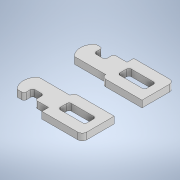
# Autodesk Inventor part: Base_modded
Saved by Autodesk Inventor 2022 (Build 260153000, 153)
## iProperties
Created: 2023-01-30
Part Number: Base_modded
Material: Generic
Document SubType Name: Modeling
Designer: scott
Density: 1 g/cm^3
Appearance: Default
Author: scott
Autodesk Inventor part; units mm, degrees
ref_plane "YZ Plane" through (0, 0, 0) normal (1, 0, 0) x (0, 1, 0)
ref_plane "XZ Plane" through (0, 0, 0) normal (0, 1, 0) x (-1, 0, 0)
ref_plane "XY Plane" through (0, 0, 0) normal (0, 0, 1) x (1, 0, 0)
sketch "Sketch1" plane through (0, 0, 0) normal (0, 1, 0) x (-1, 0, 0)
  line L0 (17.0278, 0) -> (-10.5342, 0)
  line L1 (-10.5342, 0) -> (-10.5342, -20.5)
  line L2 (-10.5342, -20.5) -> (17.0278, -20.5)
  line L3 (17.0278, -20.5) -> (17.0278, 0)
  line L4 (4.9658, -15.846) -> (-7.0342, -15.846)
  line L5 (-7.0342, -15.846) -> (-7.0342, -10.846)
  line L6 (-7.0342, -10.846) -> (4.9658, -10.846)
  line L7 (4.9658, -10.846) -> (4.9658, -15.846)
  circle A0 centre (-6.0342, -14.846) radius 1
  circle A1 centre (3.9658, -14.846) radius 1
  circle A2 centre (3.9658, -11.846) radius 1
  circle A3 centre (-6.0342, -11.846) radius 1
  circle A4 centre (-8.5342, -18.5) radius 2
  line L8 (17.0278, -20.5) -> (-8.5342, -20.5)
  line L9 (-8.5342, -20.5) -> (-8.5342, -6.2)
  line L10 (-8.5342, -6.2) -> (17.0278, -6.2)
  line L11 (17.0278, -6.2) -> (17.0278, -20.5)
  line L12 (-10.5342, -20.5) -> (7.4658, -20.5)
  line L13 (7.4658, -20.5) -> (7.4658, -17.5)
  line L14 (7.4658, -17.5) -> (-10.5342, -17.5)
  line L15 (-10.5342, -17.5) -> (-10.5342, -20.5)
  line L16 (7.4658, -17.5) -> (17.0278, -17.5)
  line L17 (17.0278, -17.5) -> (17.0278, -8)
  line L18 (17.0278, -8) -> (7.4658, -8)
  line L19 (7.4658, -8) -> (7.4658, -17.5)
  circle A5 centre (17.0278, -12.75) radius 6.5
  line L20 (17.0278, -17.5) -> (21.4649, -17.5)
  line L21 (21.4649, -17.5) -> (21.4649, -8)
  line L22 (21.4649, -8) -> (17.0278, -8)
  line L23 (17.0278, -8) -> (17.0278, -17.5)
  circle A6 centre (5.6658, -8) radius 1.8
  line L24 (18.4658, -17.5) -> (13.4658, -17.5)
  line L25 (13.4658, -17.5) -> (13.4658, -13.6692)
  line L26 (13.4658, -13.6692) -> (18.4658, -13.6692)
  line L27 (18.4658, -13.6692) -> (18.4658, -17.5)
  circle A7 centre (19.4658, -16.5) radius 1
  circle A8 centre (17.4658, -14.6692) radius 1
  circle A9 centre (14.4658, -14.6692) radius 1
  circle A10 centre (12.4658, -16.5) radius 1
  line L28 (-8.5342, -17.5) -> (-10.5342, -17.5)
  line L29 (-10.5342, -17.5) -> (-10.5342, -6.2)
  line L30 (-10.5342, -6.2) -> (-8.5342, -6.2)
  line L31 (-8.5342, -6.2) -> (-8.5342, -17.5)
  point P0 (0, 0)
  point P1 (4.9658, -11.846)
  point P2 (4.9658, -14.846)
  point P3 (3.9658, -15.846)
  point P4 (-6.0342, -15.846)
  point P5 (-7.0342, -14.846)
  point P6 (-7.0342, -11.846)
  point P7 (-6.0342, -10.846)
  point P8 (3.9658, -10.846)
  point P9 (-8.5342, -16.5)
  point P10 (-8.5342, -20.5)
  point P11 (12.4658, -17.5)
  point P12 (13.4658, -16.5)
  point P13 (13.4658, -14.6692)
  point P14 (14.4658, -13.6692)
  point P15 (17.4658, -13.6692)
  point P16 (18.4658, -14.6692)
  point P17 (18.4658, -16.5)
  point P18 (19.4658, -17.5)
  point P19 (5.6658, -6.2)
  point P20 (-10.5342, -18.5)
  dimension "d26" = 13
  dimension "d1" = 20.5
  dimension "d2" = 0
  dimension "d3" = 12
  dimension "d4" = 5
  dimension "d5" = 4.654
  dimension "d6" = 3.5
  dimension "d7" = 2
  dimension "d8" = 2
  dimension "d9" = 2
  dimension "d10" = 2
  dimension "d11" = 1
  dimension "d12" = 1
  dimension "d13" = 1
  dimension "d14" = 1
  dimension "d15" = 1
  dimension "d16" = 1
  dimension "d17" = 1
  dimension "d18" = 1
  dimension "d19" = 4
  dimension "d20" = 2
  dimension "d21" = 14.3
  dimension "d22" = 18
  dimension "d23" = 3
  dimension "d24" = 9.5
  dimension "d25" = 9.562
  dimension "d27" = 1.8
  dimension "d28" = 5
  dimension "d29" = 8.5
  dimension "d30" = 2
  dimension "d31" = 2
  dimension "d32" = 2
  dimension "d33" = 2
  dimension "d34" = 1
  dimension "d35" = 1
  dimension "d36" = 1
  dimension "d37" = 1
  dimension "d38" = 1
  dimension "d39" = 1
  dimension "d40" = 1
  dimension "d41" = 1
  constraints: 64 end point, 16 parallel, 10 centre point, 8 horizontal, 8 perpendicular, 5 point on line, 2 tangent, 1 midpoint, 3 other
  measures "d1" distance of L0.end L1.end
  measures "d2" distance from line of point (0, 0) L0
  measures "d3" distance of L4.start L4.end
  measures "d4" distance of L4.end L5.end
  measures "d5" distance between parallel lines of L2 L4
  measures "d6" distance between parallel lines of L1 L5
  measures "d7" diameter of A0
  measures "d8" diameter of A1
  measures "d9" diameter of A2
  measures "d10" diameter of A3
  measures "d11" distance from line of L4 A0.centre
  measures "d12" distance from line of L6 A3.centre
  measures "d13" distance from line of L4 A1.centre
  measures "d14" distance from line of L6 A2.centre
  measures "d15" distance from line of L7 A1.centre
  measures "d16" distance from line of A2.centre L7
  measures "d17" distance from line of L5 A0.centre
  measures "d18" distance from line of L5 A3.centre
  measures "d19" diameter of A4
  measures "d20" distance from line of L2 A4.centre
  measures "d21" distance between parallel lines of L10 L8
  measures "d22" distance of L13.end L14.end
  measures "d23" distance of L12.end L13.end
  measures "d24" distance of L18.end L13.end
  measures "d25" distance of L17.end L18.end
  measures "d27" distance from line of L19 A6.centre
  measures "d28" distance between parallel lines of L27 L25
  measures "d29" distance between parallel lines of L7 L25
  measures "d30" diameter of A7
  measures "d31" diameter of A8
  measures "d32" diameter of A9
  measures "d33" diameter of A10
  measures "d34" distance from line of L20 A7.centre
  measures "d35" distance from line of L27 A7.centre
  measures "d36" distance from line of L27 A8.centre
  measures "d37" distance from line of L26 A8.centre
  measures "d38" distance from line of L26 A9.centre
  measures "d39" distance from line of L16 A10.centre
  measures "d40" distance from line of L25 A10.centre
  measures "d41" distance from line of L25 A9.centre
extrude "Extrusion1" add sketch "Sketch1" along normal blind 3 contours L30 L9 A4 L14 L1 | A6 L19 L14 A4 L9 L10 | A6 | L14 A4 L1 | L22 L21 L20 A7 L27 L26 L3 | L3 L26 L25 A10 A5 L18 | A5 L21 | A5 A10 L16 L19 L18 | A4 L14 L9 | A4 L9 L14 | A4 L14 L9 | A10 A5 | A5 A10 | L13 L2 A4 L14 | L9 L14 A4 | A9 L25 L26 | L26 L27 A8 | A7 | L4 A1 L7 | L4 L5 A0 | A2 L6 L7 | L5 L6 A3
mirror "Mirror1" about plane through (0, 0, 0) normal (0, 0, 1) of "Extrusion1"
body "Solid1"
